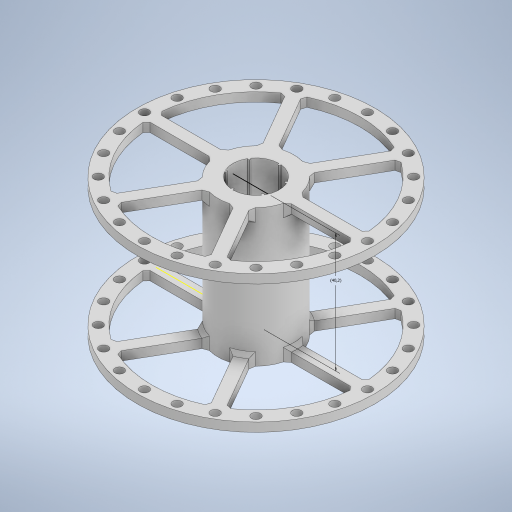
# Autodesk Inventor part: WheelV1
Saved by Autodesk Inventor 2024 (Build 280153000, 153)
## iProperties
Created: 2024-01-02
Part Number: WheelV1
Material: Generisch
Document SubType Name: Modeling
Designer: chris
Density: 1 g/cm^3
Appearance: Vorgabe
Author: chris
Autodesk Inventor part; units mm, degrees
ref_plane "YZ Plane" through (0, 0, 0) normal (1, 0, 0) x (0, 1, 0)
ref_plane "XZ Plane" through (0, 0, 0) normal (0, 1, 0) x (-1, 0, 0)
ref_plane "XY Plane" through (0, 0, 0) normal (0, 0, 1) x (1, 0, 0)
sketch "Skizze1" plane through (0, 0, 0) normal (0, 0, 1) x (1, 0, 0)
  circle A0 centre (0, 0) radius 7.75
  circle A1 centre (0, 0) radius 12.75
  dimension "d2" = 15.5
  dimension "d3" = 25.5
  constraints: 2 centre point, 1 coincident
  measures "d2" diameter of A0
  measures "d3" diameter of A1
extrude "Extrusion1" add sketch "Skizze1" along normal mid plane 46.2
sketch "Skizze3" plane through (0, 0, 23.1) normal (0, 0, 1) x (1, 0, 0)
  circle A0 centre (0, 0) radius 35
  circle A1 centre (0, 0) radius 40
  dimension "d6" = 70
  dimension "d7" = 80
  constraints: 2 centre point, 2 coincident
  measures "d6" diameter of A0
  measures "d7" diameter of A1
extrude "Extrusion2" add sketch "Skizze3" against normal blind 3
sketch "Skizze4" plane through (0, 0, 23.1) normal (0, 0, 1) x (1, 0, 0)
  circle A0 centre (0, 0) radius 12.75 construction
  circle A1 centre (0, 0) radius 35 construction
  line L0 (-12.7499, 0.05) -> (-35, 0.05)
  line L1 (-12.7499, 0.05) -> (-12.4499, 0.05) construction
  arc A2 (-12.7499, 0.05) -> (-12.7, 1.1281) centre (0, 0) ccw
  arc A3 (-35, 0.05) -> (-34.9637, 1.5937) centre (0, 0) ccw
  line L2 (-12.6, -1.95) -> (-34.9456, -1.95)
  dimension "d13" = 0.3
  dimension "d21" = 2
  constraints: 10 point on circle, 6 end point, 3 horizontal, 2 centre point, 2 concentric
  measures "d13" distance of L0.start L1.end
  measures "d21" distance between parallel lines of L0 L2
extrude "Extrusion4" add sketch "Skizze4" against normal blind 3
chamfer "Fasen1" distance 1.25 angle 45 2 edges at (-12.6, -1.95, 21.6) (-34.9456, -1.95, 21.6)
mirror "Spiegeln2" about plane through (0, 0, 0) normal (0, 1, 0) of "Extrusion4", "Fasen1"
pattern_circular "Runde Anordnung2" count 6 over 360 about axis through (0, 0, -10) along (0, 0, 1) of "Extrusion4", "Fasen1", "Spiegeln2"
chamfer "Fasen2" distance 1.25 angle 45 7 edges at (6.375, 11.0418, 20.1) (12.6492, -1.5999, 20.1) (12.6492, 1.5999, 20.1) (-6.375, 11.0418, 20.1) (6.375, -11.0418, 20.1) (-6.375, -11.0418, 20.1) (-12.75, 0, 20.1)
sketch "Skizze5" plane through (0, 0, 23.1) normal (0, 0, 1) x (1, 0, 0)
  circle A0 centre (0, 0) radius 40 construction
  line L0 (0, -40) -> (0, -35) construction
  arc A1 (-14.6585, -31.7825) -> (14.6585, -31.7825) centre (0, 0) ccw construction
  circle A2 centre (0, -37.5) radius 1.5
  dimension "d33" = 3
  constraints: 2 end point, 1 centre point, 1 midpoint, 1 point on circle, 1 vertical, 1 vertical alignment, 1 other
  measures "d33" diameter of A2
extrude "Extrusion5" cut sketch "Skizze5" against normal blind 3
pattern_circular "Runde Anordnung3" count 24 over 360 about axis through (0, 0, -10) along (0, 0, 1) of "Extrusion5"
mirror "Spiegeln3" about plane through (0, 0, 0) normal (0, 0, 1) of "Extrusion4", "Fasen1", "Spiegeln2", "Runde Anordnung2", "Extrusion2", "Extrusion5", "Runde Anordnung3", "Fasen2"
sketch "Skizze6" plane through (0, 0, 0) normal (0, 0, 1) x (1, 0, 0)
  circle A0 centre (0, 0) radius 7.75 projected
  line L0 (0, 7.75) -> (0, 7.12)
  line L1 (0, 7.12) -> (0.75, 7.12)
  line L2 (0.75, 7.12) -> (0.75, 7.7136)
  arc A1 (0.75, 7.7136) -> (1.464, 7.6105) centre (0, 0) ccw
  dimension "d39" = 0.63
  dimension "d40" = 0.75
  constraints: 6 end point, 6 point on circle, 2 vertical, 1 centre point, 1 concentric, 1 perpendicular
  measures "d39" distance of L0.start L0.end
  measures "d40" distance of L0.end L1.end
extrude "Extrusion6" add sketch "Skizze6" along normal mid plane 46.2 contours A0 L2 L1 L0 picked at (0.4168, 7.3246)
pattern_circular "Runde Anordnung4" count 6 over 360 about axis through (0, 0, -10) along (0, 0, 1) of "Extrusion6"
fillet "Rundung1" radius 0.35 12 edges at (6.1661, 3.56, 0) (6.5411, 2.9105, 0) (6.1661, -3.56, 0) (5.7911, -4.2095, 0) (0.75, 7.12, 0) (0, 7.12, 0) (-6.1661, 3.56, 0) (-5.7911, 4.2095, 0) (-6.5411, -2.9105, 0) (-6.1661, -3.56, 0) (0, -7.12, 0) (-0.75, -7.12, 0)
sketch "Skizze7" plane through (0, 0, 0) normal (0, 1, 0) x (-1, 0, 0)
  line L0 (16.2884, 20.1) -> (-4.6281, 20.1)
  line L1 (14.6585, 20.1) -> (-14.6585, 20.1) projected
  line L2 (13.8635, -20.1) -> (33.6956, -20.1) projected
  line L3 (17.9713, -20.1) -> (-2.3441, -20.1)
  point P0 (0, 0)
  dimension "d47" = 40.2
  constraints: 4 end point, 2 point on line, 1 collinear
  measures "d47" distance between parallel lines of L3 L0
